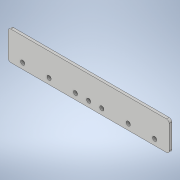
# Autodesk Inventor part: 20220523_センサモジュール
Saved by Autodesk Inventor 2020 (Build 240168000, 168)
## iProperties
Created: 2021-05-16
Part Number: 20220523_センサモジュール
Material: 一般
Document SubType Name: Modeling
Designer: fmasa
Density: 1 g/cm^3
Appearance: 既定
Mass: 5.24854 g
Surface Area: 59.5841 cm^2
Volume: 5.24854 cm^3
Author: fmasa
Autodesk Inventor part; units mm, degrees
ref_plane "YZ Plane" through (0, 0, 0) normal (1, 0, 0) x (0, 1, 0)
ref_plane "XZ Plane" through (0, 0, 0) normal (0, 1, 0) x (-1, 0, 0)
ref_plane "XY Plane" through (0, 0, 0) normal (0, 0, 1) x (1, 0, 0)
sketch "スケッチ1" plane through (0, 0, 0) normal (0, 0, 1) x (1, 0, 0)
  line L0 (2, 0) -> (120, 0)
  line L1 (122, 2) -> (122, 20)
  line L2 (120, 22) -> (2, 22)
  line L3 (0, 20) -> (0, 2)
  circle A0 centre (11, 4.5) radius 1.6
  circle A1 centre (31, 4.5) radius 1.6
  circle A2 centre (51, 4.5) radius 1.6
  line L4 (61, 33.5385) -> (61, -12.997) construction
  circle A3 centre (61, 4.5) radius 1.6
  line L5 (-8.4067, 4.5) -> (129.3386, 4.5) construction
  circle A4 centre (111, 4.5) radius 1.6
  circle A5 centre (91, 4.5) radius 1.6
  circle A6 centre (71, 4.5) radius 1.6
  arc A7 (2, 22) -> (0, 20) centre (2, 20) ccw
  arc A8 (0, 2) -> (2, 0) centre (2, 2) ccw
  arc A9 (120, 0) -> (122, 2) centre (120, 2) ccw
  arc A10 (122, 20) -> (120, 22) centre (120, 20) ccw
  point P0 (0, 0)
  point P1 (122, 22)
  point P2 (122, 0)
  point P3 (0, 22)
  dimension "d0" = 122
  dimension "d1" = 22
  dimension "d2" = 3.2
  dimension "d3" = 3.2
  dimension "d4" = 3.2
  dimension "d5" = 10
  dimension "d6" = 20
  dimension "d7" = 20
  dimension "d8" = 3.2
  dimension "d9" = 4.5
  dimension "d10" = 2
  constraints: 13 point on line, 12 end point, 11 centre point, 8 point on circle, 8 tangent, 3 equal radius, 3 symmetric about line, 2 horizontal, 2 parallel, 1 perpendicular, 1 vertical, 4 other
  measures "d0" distance of point (0, 22) point (122, 22)
  measures "d1" distance of point (122, 22) point (122, 0)
  measures "d2" diameter of A0
  measures "d3" diameter of A1
  measures "d4" diameter of A2
  measures "d5" distance from line of L4 A2.centre
  measures "d6" distance of A2.centre A1.centre
  measures "d7" distance of A1.centre A0.centre
  measures "d8" diameter of A3
  measures "d9" distance between parallel lines of L5 L0
  measures "d10" radius of A7
extrude "押し出し1" add sketch "スケッチ1" along normal blind 2
